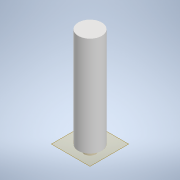
# Autodesk Inventor part: motor_1.0
Saved by Autodesk Inventor 2020 (Build 240168000, 168)
## iProperties
Created: 2020-07-03
Part Number: motor_1.0
Material: Generic
Document SubType Name: Modeling
Designer: Ashiqrahman
Density: 1 g/cm^3
Appearance: Default
Author: Ashiqrahman
Autodesk Inventor part; units mm, degrees
ref_plane "YZ Plane" through (0, 0, 0) normal (1, 0, 0) x (0, 1, 0)
ref_plane "XZ Plane" through (0, 0, 0) normal (0, 1, 0) x (-1, 0, 0)
ref_plane "XY Plane" through (0, 0, 0) normal (0, 0, 1) x (1, 0, 0)
ref_plane "Work Plane1" through (99.4239, 56.7932, 22.5839) normal (0, 1, 0) x (-1, 0, 0)
sketch "Sketch1" plane through (99.4239, 56.7932, 22.5839) normal (0, 1, 0) x (-1, 0, 0)
  arc A0 (3.8626, -3.175) -> (-3.8626, -3.175) centre (0, 0) ccw projected
  line L0 (3.8626, -3.175) -> (-3.8626, -3.175) projected
  circle A1 centre (0, 0) radius 7.5 projected
  circle A2 centre (0, 0) radius 10 projected
  point P0 (99.4239, -22.5839)
extrude "Extrusion1" add sketch "Sketch1" along normal blind 85.0001 contours L0 A0 | A1 | A2
sketch "Sketch2" plane through (99.4239, 56.7932, 22.5839) normal (0, -1, 0) x (1, 0, 0)
  line L0 (-3.8626, -3.175) -> (3.8626, -3.175) projected
  arc A0 (3.8626, -3.175) -> (-3.8626, -3.175) centre (0, 0) ccw projected
  point P0 (-99.4239, -22.5839)
extrude "Extrusion2" add sketch "Sketch2" along normal blind 5
body "Solid1"
